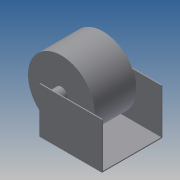
# Autodesk Inventor part: winch
Saved by Autodesk Inventor 2013 SP2 (Build 170200200, 200)
## iProperties
Created: 2013-12-16
Part Number: winch
Material: Generic
Document SubType Name: Modeling
Designer: Dave
Density: 1 g/cm^3
Author: Dave
Autodesk Inventor part; units mm, degrees
ref_plane "YZ Plane" through (0, 0, 0) normal (1, 0, 0) x (0, 1, 0)
ref_plane "XZ Plane" through (0, 0, 0) normal (0, 1, 0) x (-1, 0, 0)
ref_plane "XY Plane" through (0, 0, 0) normal (0, 0, 1) x (1, 0, 0)
sketch "Sketch1" plane through (0, 0, 0) normal (0, 0, 1) x (1, 0, 0)
  circle A0 centre (0, 0) radius 50.8
  dimension "d0" = 101.6
  constraints: 1 centre point, 1 coincident
  measures "d0" diameter of A0
extrude "Extrusion1" add sketch "Sketch1" along normal blind 63.5
sketch "Sketch2" plane through (0, 0, 63.5) normal (0, 0, 1) x (1, 0, 0)
  circle A0 centre (0, 0) radius 50.8 projected
  circle A1 centre (0, 0) radius 9.525
  dimension "d5" = 19.05
  constraints: 1 centre point, 1 coincident
  measures "d5" diameter of A1
extrude "Extrusion2" add sketch "Sketch2" along normal blind 15.875 and the other way blind 76.2 contours A1
sketch "Sketch3" plane through (0, 0, 79.375) normal (0, 0, 1) x (1, 0, 0)
  line L0 (-15.875, -55.5625) -> (79.375, -55.5625)
  line L1 (79.375, -55.5625) -> (79.375, 14.2875)
  line L2 (79.375, 14.2875) -> (-15.875, 14.2875)
  line L3 (-15.875, 14.2875) -> (-15.875, -55.5625)
  dimension "d11" = 95.25
  dimension "d13" = 69.85
  constraints: 8 end point, 2 parallel, 1 horizontal, 1 perpendicular
  measures "d11" distance of L0.start L0.end
  measures "d13" distance of L2.end L0.start
extrude "Extrusion3" add sketch "Sketch3" along normal blind 1.524
sketch "Sketch4" plane through (0, 0, 79.375) normal (0, 0, -1) x (-1, 0, 0)
  line L0 (15.875, -55.5625) -> (-79.375, -55.5625) projected
  line L1 (15.875, 14.2875) -> (15.875, -55.5625) projected
  line L2 (-79.375, -55.5625) -> (15.875, -55.5625)
  line L3 (15.875, -55.5625) -> (15.875, -54.0385)
  line L4 (15.875, -54.0385) -> (-79.375, -54.0385)
  line L5 (-79.375, -54.0385) -> (-79.375, -55.5625)
  dimension "d16" = 1.524
  constraints: 8 end point, 2 parallel, 1 horizontal, 1 perpendicular, 1 point on line
  measures "d16" distance of L4.end L0.end
extrude "Extrusion4" add sketch "Sketch4" along normal blind 88.9
sketch "Sketch5" plane through (0, 0, -9.525) normal (0, 0, -1) x (-1, 0, 0)
  line L0 (-79.375, -55.5625) -> (15.875, -55.5625)
  line L1 (15.875, -55.5625) -> (15.875, 14.2875)
  line L2 (15.875, 14.2875) -> (-79.375, 14.2875)
  line L3 (-79.375, 14.2875) -> (-79.375, -55.5625)
  point P0 (0, 0)
  constraints: 8 end point, 2 parallel, 1 horizontal, 1 perpendicular
extrude "Extrusion5" add sketch "Sketch5" along normal blind 1.524
body "Solid1"
